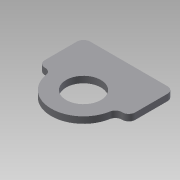
# Autodesk Inventor part: Гор. шарнир
Saved by Autodesk Inventor 2018 (Build 220112000, 112)
## iProperties
Created: 2020-02-22
Part Number: Гор. шарнир
Material: Типовые
Document SubType Name: Modeling
Designer: Leancher
Density: 1 g/cm^3
Appearance: По умолчанию
Author: Leancher
Autodesk Inventor part; units mm, degrees
ref_plane "YZ Plane" through (0, 0, 0) normal (1, 0, 0) x (0, 1, 0)
ref_plane "XZ Plane" through (0, 0, 0) normal (0, 1, 0) x (-1, 0, 0)
ref_plane "XY Plane" through (0, 0, 0) normal (0, 0, 1) x (1, 0, 0)
sketch "Эскиз1" plane through (0, 0, 0) normal (0, 0, 1) x (1, 0, 0)
  line L0 (29.9986, 35) -> (-30, 35)
  arc A0 (-30, 35) -> (-35, 30) centre (-30, 30) ccw
  line L1 (-35, 30) -> (-35, 5)
  arc A1 (-35, 5) -> (-30, 0) centre (-30, 5) ccw
  line L2 (-30, 0) -> (-29.5804, 0)
  arc A2 (-24.6503, -4.1667) -> (-29.5804, 0) centre (-29.5804, -5) ccw
  arc A3 (-24.6503, -4.1667) -> (24.6503, -4.1667) centre (0, 0) ccw
  arc A4 (29.5804, 0) -> (24.6503, -4.1667) centre (29.5804, -5) ccw
  arc A5 (29.5804, 0) -> (34.9985, 4.9825) centre (29.9985, 4.9825) ccw
  line L3 (34.9985, 4.9825) -> (34.9985, 29.9825)
  arc A6 (34.9985, 29.9825) -> (29.9986, 35) centre (29.9986, 30) ccw
  circle A7 centre (0, 0) radius 13.45
  line L4 (-0.0007, 35) -> (-0.0007, -40.0249) construction
  line L5 (-31.1692, 11.8598) -> (-24.8192, 11.8598)
  line L6 (-24.8192, 11.8598) -> (-24.8192, 31.7098)
  line L7 (-24.8192, 31.7098) -> (-31.1692, 31.7098)
  line L8 (-31.1692, 31.7098) -> (-31.1692, 11.8598)
  line L9 (24.8177, 11.8598) -> (31.1677, 11.8598)
  line L10 (31.1677, 11.8598) -> (31.1677, 31.7098)
  line L11 (31.1677, 31.7098) -> (24.8177, 31.7098)
  line L12 (24.8177, 31.7098) -> (24.8177, 11.8598)
  point P0 (29.9986, 30)
  point P1 (-30, 30)
  point P2 (25.9869, 30)
  constraints: 26 end point, 14 point on circle, 8 centre point, 1 midpoint, 1 symmetric about line, 1 vertical
extrude "Выдавливание1" add sketch "Эскиз1" along normal blind 5
